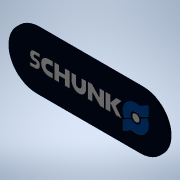
# Autodesk Inventor part: SCHUNK-9954530 Typenschild 6x17x0.3
Saved by Autodesk Inventor 2021 (Build 250183000, 183)
## iProperties
Created: 2025-07-30
Part Number: SCHUNK-9954530 Typenschild 6x17x0.3
Material: Generic
Catalog Web Link: www.cadenas.de
Description: Typenschild-SCHUNK-Typenschild
Vendor: SCHUNK
Document SubType Name: Modeling
Designer: psAdmin
Manufacturer: SCHUNK
Mass: 0.0274526 g
Surface Area: 2.04217 cm^2
Volume: 0.0274526 cm^3
Density: 1 g/cm^3
Appearance: PSOLRGB-175-175-175
Category: PARTsolutions
Company: SCHUNK
Title: SCHUNK-9954530 Typenschild 6x17x0.3
Author: Cadenas PARTsolutions
Comments: SCHUNK-Typenschild
PSOL_IDENT_0: {$CADENAS_DATA/23d-libs/schunk/normteile/typenschilder.prj},215 {VTYP=3D},{NB=SCHUNK-9954530 Typensc
PSOL_IDENT_1: hild 6x17x0.3},{LINA=SCHUNK-9954530 Typenschild 6x17x0.3},{NN=Typenschild},{DATE=28.01.2025 09:52:53
PSOL_IDENT_2: },{GEOMDATE=05.06.2024 07:11:39},{VERSION=},{LINEID=30},{WBVAR=},{WBNUMERIC=}  {NB=SCHUNK-9954530 Ty
PSOL_IDENT_3: penschild 6x17x0.3},{LINA=SCHUNK-9954530 Typenschild 6x17x0.3},{KT=DUMMY},{IDNR=9954530},{TYP=6x17x0
PSOL_IDENT_4: .3},{B=6.000},{L=17.000},{H=0.300},{SF=2.200},{SFL=1.650},{SFS=0.145},{SFBS=1.750},{VBS=-0.025},{VBC=
PSOL_IDENT_5: -0.080},{VBU=-0.045},{VL=5.000},{VS=-35.950},{TYP1=3.000},{PARTSERVER=1.000}
NB: SCHUNK-9954530 Typenschild 6x17x0.3
NN: Typenschild
NT: SCHUNK-Typenschild
NBSYN: SCHUNK-$IDNR. Typenschild $TYP.
LINA: SCHUNK-9954530 Typenschild 6x17x0.3
CATALOG: SCHUNK
IDNR: 9954530
TYP: 6x17x0.3
B: 6
L: 17
H: 0.3
SF: 2.2
SFL: 1.65
SFS: 0.145
SFBS: 1.75
VBS: -0.025
VBC: -0.08
VBU: -0.045
VL: 5
VS: -35.95
TYP1: 3
PARTSERVER: 1
SUPPLIER: SCHUNK
ARTICLENO: SCHUNK-9954530 Typenschild 6x17x0.3
BOMINFO: SCHUNK-9954530 Typenschild 6x17x0.3
CREATOR: CADENAS GmbH
Autodesk Inventor part; units mm, degrees
sketch "Sketch_1" plane through (0, 0, 0) normal (0, 0, 1) x (1, 0, 0)
  arc A0 (-8.5, 0) -> (-5.5, -3) centre (-5.5, 0) ccw
  line L0 (-5.5, -3) -> (5.5, -3)
  arc A1 (5.5, -3) -> (8.5, 0) centre (5.5, 0) ccw
  arc A2 (8.5, 0) -> (5.5, 3) centre (5.5, 0) ccw
  line L1 (5.5, 3) -> (-5.5, 3)
  arc A3 (-5.5, 3) -> (-8.5, 0) centre (-5.5, 0) ccw
  constraints: 8 point on circle, 4 centre point, 4 end point
extrude "Extrusion1" add sketch "Sketch_1" along normal blind 0.3
sketch "Sketch_13" plane through (0, 0, 0.3) normal (0, 0, 1) x (1, 0, 0)
  line L0 (-3.6632, 0.8041) -> (-3.6632, -0.8054)
  line L1 (-3.6632, -0.8054) -> (-3.1273, -0.8054)
  line L2 (-3.1273, -0.8054) -> (-3.1273, -0.1965)
  line L3 (-3.1273, -0.1965) -> (-2.5376, -0.1965)
  line L4 (-2.5376, -0.1965) -> (-2.5376, -0.8054)
  line L5 (-2.5376, -0.8054) -> (-2.0015, -0.8054)
  line L6 (-2.0015, -0.8054) -> (-2.0015, 0.8041)
  line L7 (-2.0015, 0.8041) -> (-2.5376, 0.8041)
  line L8 (-2.5376, 0.8041) -> (-2.5376, 0.2189)
  line L9 (-2.5376, 0.2189) -> (-3.1273, 0.2189)
  line L10 (-3.1273, 0.2189) -> (-3.1273, 0.8041)
  line L11 (-3.1273, 0.8041) -> (-3.6632, 0.8041)
  constraints: 24 end point
extrude "Extrusion2" cut sketch "Sketch_13" against normal blind 0.05
sketch "Sketch_15" plane through (0, 0, 0.3) normal (0, 0, 1) x (1, 0, 0)
  line L0 (-0.1071, 0.8041) -> (-0.1071, -0.8054)
  line L1 (-0.1071, -0.8054) -> (0.4065, -0.8054)
  line L2 (0.4065, -0.8054) -> (0.4065, 0.0207)
  line L3 (0.4065, 0.0207) -> (1.1802, -0.8054)
  line L4 (1.1802, -0.8054) -> (1.6375, -0.8054)
  line L5 (1.6375, -0.8054) -> (1.6375, 0.8041)
  line L6 (1.6375, 0.8041) -> (1.1241, 0.8041)
  line L7 (1.1241, 0.8041) -> (1.1241, -0.0218)
  line L8 (1.1241, -0.0218) -> (0.3505, 0.8041)
  line L9 (0.3505, 0.8041) -> (-0.1071, 0.8041)
  constraints: 20 end point
extrude "Extrusion3" cut sketch "Sketch_15" against normal blind 0.05
sketch "Sketch_16" plane through (0, 0, 0.3) normal (0, 0, 1) x (1, 0, 0)
  line L0 (1.7754, 0.8041) -> (1.7754, -0.8054)
  line L1 (1.7754, -0.8054) -> (2.3114, -0.8054)
  line L2 (2.3114, -0.8054) -> (2.3114, -0.0465)
  line L3 (2.3114, -0.0465) -> (2.8699, -0.8054)
  line L4 (2.8699, -0.8054) -> (3.5089, -0.8054)
  line L5 (3.5089, -0.8054) -> (2.8629, 0.0559)
  line L6 (2.8629, 0.0559) -> (3.4864, 0.8041)
  line L7 (3.4864, 0.8041) -> (2.9235, 0.8041)
  line L8 (2.9235, 0.8041) -> (2.3114, 0.0749)
  line L9 (2.3114, 0.0749) -> (2.3114, 0.8041)
  line L10 (2.3114, 0.8041) -> (1.7754, 0.8041)
  constraints: 22 end point
extrude "Extrusion4" cut sketch "Sketch_16" against normal blind 0.05
sketch "Sketch_5" plane through (0, 0, 0.3) normal (0, 0, 1) x (1, 0, 0)
  arc A0 (-6.2375, 0.1925) -> (-5.8875, -0.1575) centre (-5.8875, 0.1925) ccw
  line L0 (-5.8875, -0.1575) -> (-5.7038, -0.1575)
  arc A1 (-5.7038, -0.455) -> (-5.7038, -0.1575) centre (-5.7038, -0.3063) ccw
  line L1 (-5.7038, -0.455) -> (-6.2375, -0.455)
  line L2 (-6.2375, -0.455) -> (-6.2375, -0.7875)
  line L3 (-6.2375, -0.7875) -> (-5.6775, -0.7875)
  arc A2 (-5.6775, -0.7875) -> (-5.1875, -0.2975) centre (-5.6775, -0.2975) ccw
  line L4 (-5.1875, -0.2975) -> (-5.1875, -0.1925)
  arc A3 (-5.1875, -0.1925) -> (-5.5375, 0.1575) centre (-5.5375, -0.1925) ccw
  line L5 (-5.5375, 0.1575) -> (-5.7038, 0.1575)
  arc A4 (-5.7038, 0.455) -> (-5.7038, 0.1575) centre (-5.6991, 0.3063) ccw
  line L6 (-5.7038, 0.455) -> (-5.1875, 0.455)
  line L7 (-5.1875, 0.455) -> (-5.1875, 0.7875)
  line L8 (-5.1875, 0.7875) -> (-5.7475, 0.7875)
  arc A5 (-5.7475, 0.7875) -> (-6.2375, 0.2975) centre (-5.7475, 0.2975) ccw
  line L9 (-6.2375, 0.2975) -> (-6.2375, 0.1925)
  constraints: 20 end point, 12 point on circle, 6 centre point
extrude "Extrusion5" cut sketch "Sketch_5" against normal blind 0.05
sketch "Sketch_6" plane through (0, 0, 0.3) normal (0, 0, 1) x (1, 0, 0)
  arc A0 (-4.28, 0.7963) -> (-4.28, -0.7963) centre (-4.28, 0) ccw
  line L0 (-4.28, -0.7963) -> (-3.825, -0.7963)
  line L1 (-3.825, -0.7963) -> (-3.825, -0.2975)
  line L2 (-3.825, -0.2975) -> (-4.28, -0.2975)
  arc A1 (-4.28, 0.2975) -> (-4.28, -0.2975) centre (-4.28, 0) ccw
  line L3 (-4.28, 0.2975) -> (-3.825, 0.2975)
  line L4 (-3.825, 0.2975) -> (-3.825, 0.7963)
  line L5 (-3.825, 0.7963) -> (-4.28, 0.7963)
  constraints: 12 end point, 4 point on circle, 2 centre point
extrude "Extrusion6" cut sketch "Sketch_6" against normal blind 0.05
sketch "Sketch_7" plane through (0, 0, 0.3) normal (0, 0, 1) x (1, 0, 0)
  line L0 (-1.845, 0.77) -> (-1.845, 0)
  arc A0 (-1.845, 0) -> (-0.27, 0) centre (-1.0575, 0) ccw
  line L1 (-0.27, 0) -> (-0.27, 0.77)
  line L2 (-0.27, 0.77) -> (-0.7775, 0.77)
  line L3 (-0.7775, 0.77) -> (-0.7775, 0)
  arc A1 (-1.3375, 0) -> (-0.7775, 0) centre (-1.0575, 0) ccw
  line L4 (-1.3375, 0) -> (-1.3375, 0.77)
  line L5 (-1.3375, 0.77) -> (-1.845, 0.77)
  constraints: 12 end point, 4 point on circle, 2 centre point
extrude "Extrusion7" cut sketch "Sketch_7" against normal blind 0.05
sketch "Sketch8" plane through (0, 0, 0.3) normal (0, 0, 1) x (1, 0, 0)
  point P0 (5, 0)
hole "Hole1" at (5, 0, 0.3) direction (0, 0, -1) diameter 0.792 depth 0.05
sketch "Sketch_3" plane through (0, 0, 0.3) normal (0, 0, 1) x (1, 0, 0)
  arc A0 (5.4071, 1.3376) -> (3.7386, -0.6031) centre (5, 0) ccw
  line L0 (3.7386, -0.6031) -> (4.491, -0.2074)
  arc A1 (5.4546, 0.309) -> (4.491, -0.2074) centre (5, 0) ccw
  line L1 (5.4546, 0.309) -> (6.3827, 0.8023)
  line L2 (6.3827, 0.8023) -> (6.3827, 1.855)
  line L3 (6.3827, 1.855) -> (5.4071, 1.3376)
  constraints: 8 end point, 4 point on circle, 2 centre point
extrude "Extrusion8" cut sketch "Sketch_3" against normal blind 0.05
sketch "Sketch_4" plane through (0, 0, 0.3) normal (0, 0, 1) x (1, 0, 0)
  line L0 (3.6223, -0.799) -> (3.6223, -1.8517)
  line L1 (3.6223, -1.8517) -> (4.5982, -1.3386)
  arc A0 (4.5982, -1.3386) -> (6.258, 0.6089) centre (5, 0) ccw
  line L2 (6.258, 0.6089) -> (5.5078, 0.205)
  arc A1 (4.5487, -0.3102) -> (5.5078, 0.205) centre (5, 0) ccw
  line L3 (4.5487, -0.3102) -> (3.6223, -0.799)
  constraints: 8 end point, 4 point on circle, 2 centre point
extrude "Extrusion9" cut sketch "Sketch_4" against normal blind 0.05
ref_plane "aluschild_XY" through (0, 0, 0) normal (0, 0, 1) x (1, 0, 0)
ref_plane "aluschild_YZ" through (0, 0, 0) normal (1, 0, 0) x (0, 1, 0)
ref_plane "aluschild_ZX" through (0, 0, 0) normal (0, 1, 0) x (0, 0, 1)
body "Solid1"
